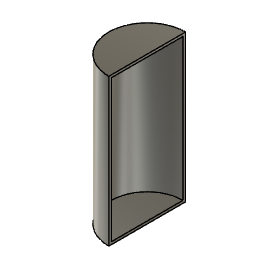
can v3 v1 (Autodesk Fusion 360 design; units mm, degrees)
Autodesk Fusion 360 part; units mm, degrees
sketch "Sketch2" plane through (0, 0, 0) normal (1, 0, 0) x (0, 1, 0)
  line L0 (0, 0) -> (30, 0)
  line L1 (30, 0) -> (30, 115)
  line L2 (30, 115) -> (0, 115)
  line L3 (0, 2) -> (28, 2)
  line L4 (28, 2) -> (28, 113)
  line L5 (28, 113) -> (0, 113)
  line L6 (0, 113) -> (0, 115)
  line L7 (0, 2) -> (0, 0)
  dimension "d2" = 30
  dimension "d3" = 115
  dimension "d4" = -2
  constraint coincident L0.start L7.end
  constraint horizontal L0
  constraint perpendicular L0 L1
  constraint perpendicular L1 L2
  constraint perpendicular L2 L6
  constraint perpendicular L0 L7
  measures "d2" distance of L0.start L0.end
  measures "d3" distance of L0.end L1.end
revolve "Revolve1" add sketch "Sketch2" angle 360 about axis through (0, 0, 1.75) along (0, 0, 1) makes body 1
split "Split1" by plane through (0, 0, 0) normal (1, 0, 0) bodies 1 makes body 2 at (2.987, 29.8509, 76.6667)
hidden bodies 2
